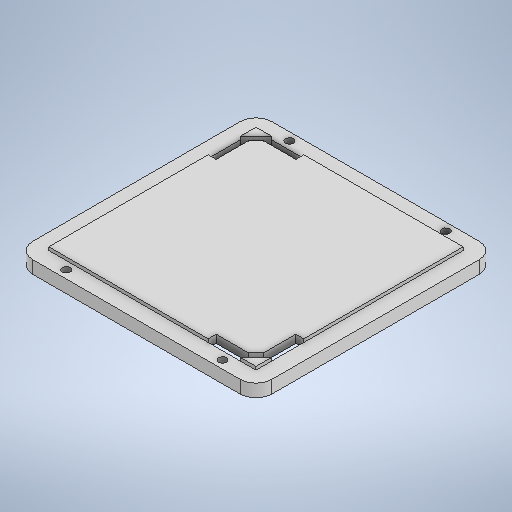
# Autodesk Inventor part: Tampa
Saved by Autodesk Inventor 2025.2 (Build 292293000, 293)
## iProperties
Created: 2025-03-23
Part Number: Tampa
Material: Genérico
Document SubType Name: Modeling
Designer: miche
Density: 1 g/cm^3
Appearance: Padrão
Author: miche
Autodesk Inventor part; units mm, degrees
ref_plane "YZ Plane" through (0, 0, 0) normal (1, 0, 0) x (0, 1, 0)
ref_plane "XZ Plane" through (0, 0, 0) normal (0, 1, 0) x (-1, 0, 0)
ref_plane "XY Plane" through (0, 0, 0) normal (0, 0, 1) x (1, 0, 0)
sketch "Esboço1" plane through (0, 0, 0) normal (0, 1, 0) x (-1, 0, 0)
  line L0 (5, 0) -> (70, 0)
  line L1 (75, -5) -> (75, -70)
  line L2 (70, -75) -> (5, -75)
  line L3 (0, -70) -> (0, -5)
  arc A0 (70, -75) -> (75, -70) centre (70, -70) ccw
  arc A1 (0, -70) -> (5, -75) centre (5, -70) ccw
  arc A2 (75, -5) -> (70, 0) centre (70, -5) ccw
  arc A3 (5, 0) -> (0, -5) centre (5, -5) ccw
  point P0 (0, 0)
  point P1 (75, -75)
  point P2 (75, 0)
  point P3 (0, -75)
  dimension "d0" = 75
  dimension "d1" = 75
  dimension "d2" = 5
  constraints: 8 end point, 8 point on circle, 8 point on line, 8 tangent, 4 centre point, 3 equal radius, 2 parallel, 1 horizontal, 1 perpendicular
  measures "d0" distance of point (75, -75) point (0, -75)
  measures "d1" distance of point (75, 0) point (75, -75)
  measures "d2" radius of A0
extrude "Extrusão1" add sketch "Esboço1" along normal blind 5
sketch "Esboço2" plane through (0, 5, 0) normal (0, 1, 0) x (1, 0, 0)
  line L0 (0, 75) -> (-13, 75)
  line L1 (-75, 75) -> (-62, 75)
  line L2 (-75, 0) -> (-62, 0)
  line L3 (-70, 0) -> (-5, 0) projected
  line L4 (0, 0) -> (-13, 0)
  line L5 (-13, 75) -> (-13, 72.5)
  line L6 (-62, 75) -> (-62, 72.5)
  line L7 (-62, 0) -> (-62, 2.5)
  line L8 (-13, 0) -> (-13, 2.5)
  circle A0 centre (-62, 72.5) radius 1.25
  circle A1 centre (-13, 72.5) radius 1.25
  circle A2 centre (-62, 2.5) radius 1.25
  circle A3 centre (-13, 2.5) radius 1.25
  dimension "d5" = 13
  dimension "d6" = 2.5
  dimension "d7" = 2.5
  dimension "d8" = 2.5
  dimension "d9" = 2.5
  dimension "d10" = 2.5
  dimension "d11" = 2.5
  constraints: 16 end point, 4 centre point, 4 coincident, 3 point on line, 3 vertical, 1 horizontal
  measures "d5" distance of L1.start L1.end
  measures "d6" distance of L0.end L5.end
  measures "d7" distance of L2.end L7.end
  measures "d8" diameter of A0
  measures "d9" diameter of A1
  measures "d10" diameter of A2
  measures "d11" diameter of A3
extrude "Extrusão2" cut sketch "Esboço2" against normal through all
sketch "Esboço3" plane through (0, 0, 0) normal (0, -1, 0) x (1, 0, 0)
  line L0 (-5, -75) -> (-70, -75) projected
  line L1 (-5, -75) -> (-5, -70)
  line L2 (-5, -70) -> (-70, -70)
  line L3 (-70, -70) -> (-70, -5)
  line L4 (-70, -5) -> (-5, -5)
  line L5 (-5, -5) -> (-5, -70)
  point P0 (0, 0)
  dimension "d14" = 5
  dimension "d15" = 65
  dimension "d16" = 65
  constraints: 10 end point, 2 parallel, 1 horizontal, 1 perpendicular, 1 vertical
  measures "d14" distance of L0.start L1.end
  measures "d15" distance of L3.end L4.end
  measures "d16" distance of L2.end L3.end
extrude "Extrusão3" cut sketch "Esboço3" against normal blind 2.5
sketch "Esboço4" plane through (0, 5, 0) normal (0, 1, 0) x (1, 0, 0)
  line L0 (-5, 70) -> (-70, 70) projected
  line L1 (-70, 70) -> (-65, 70)
  line L2 (-70, 70) -> (-70, 65)
  line L3 (-70, 65) -> (-65, 70)
  line L4 (-70, 5) -> (-5, 5) projected
  line L5 (-5, 5) -> (-5, 10)
  line L6 (-5, 5) -> (-5, 70) projected
  line L7 (-5, 5) -> (-10, 5)
  line L8 (-10, 5) -> (-5, 10)
  line L9 (-70, 65) -> (-70, 55)
  line L10 (-70, 70) -> (-70, 5) projected
  line L11 (-70, 55) -> (-67.5, 55)
  line L12 (-65, 70) -> (-55, 70)
  line L13 (-55, 70) -> (-55, 67.5)
  line L14 (-55, 67.5) -> (-63.9645, 67.5)
  line L15 (-65, 70) -> (-55, 70)
  line L16 (-70, 65) -> (-70, 55)
  line L17 (-67.5, 65) -> (-65, 67.5)
  line L18 (-67.5, 65) -> (-67.5, 55)
  line L19 (-65, 67.5) -> (-63.9645, 67.5)
  point P0 (0, 0)
  constraints: 32 end point, 5 point on line, 3 vertical, 2 horizontal, 2 perpendicular, 1 collinear
sketch "Esboço5" plane through (0, 5, 0) normal (0, 1, 0) x (1, 0, 0)
  line L0 (-5, 5) -> (-5, 70) projected
  line L1 (-5, 10) -> (-5, 20)
  line L2 (-5, 20) -> (-7.5, 20)
  line L3 (-70, 5) -> (-5, 5) projected
  line L4 (-10, 5) -> (-20, 5)
  line L5 (-20, 5) -> (-20, 7.5)
  line L6 (-7.5, 10) -> (-10, 7.5)
  line L7 (-7.5, 20) -> (-7.5, 10)
  line L8 (-20, 7.5) -> (-10, 7.5)
  line L9 (-5, 20) -> (-5, 10)
  line L10 (-20, 5) -> (-10, 5)
  line L11 (-10, 5) -> (-5, 10)
  point P0 (0, 0)
  dimension "d23" = 2.5
  dimension "d24" = 10
  dimension "d25" = 2.5
  constraints: 20 end point, 4 point on line, 3 perpendicular, 1 collinear, 1 vertical
  measures "d23" distance of L1.end L2.end
  measures "d24" distance of L4.start L4.end
  measures "d25" distance of L4.end L5.end
extrude "Extrusão4" cut sketch "Esboço5" against normal through all contours L11 L3 L5 L8 L6 L7 L2 L0
extrude "Extrusão5" cut sketch "Esboço4" against normal through all contours L13 L14 L19 L17 L18 L11 L9 L3 L0
sketch "Esboço6" plane through (0, 5, 0) normal (0, 1, 0) x (1, 0, 0)
  line L0 (-70, 70) -> (-70, 5) projected
  line L1 (-5, 5) -> (-5, 70) projected
  line L2 (-70, 70) -> (-5, 70)
  line L3 (-5, 70) -> (-5, 5)
  line L4 (-5, 5) -> (-70, 5)
  line L5 (-70, 5) -> (-70, 70)
  arc A0 (0, 70) -> (-5, 75) centre (-5, 70) ccw projected
  line L6 (-5, 75) -> (0, 75)
  line L7 (0, 75) -> (0, 0)
  line L8 (0, 0) -> (-5, 0)
  line L9 (-5, 0) -> (-5, 75)
  line L10 (-75, 75) -> (0, 75)
  line L11 (0, 75) -> (0, 70)
  line L12 (0, 70) -> (-75, 70)
  line L13 (-75, 70) -> (-75, 75)
  line L14 (0, 0) -> (-75, 0)
  line L15 (-75, 0) -> (-75, 5)
  line L16 (-75, 5) -> (0, 5)
  line L17 (0, 5) -> (0, 0)
  line L18 (-75, 0) -> (-70, 0)
  line L19 (-70, 0) -> (-70, 75)
  line L20 (-70, 75) -> (-75, 75)
  line L21 (-75, 75) -> (-75, 0)
  constraints: 40 end point, 10 parallel, 6 point on line, 5 horizontal, 5 perpendicular
extrude "Extrusão6" cut sketch "Esboço6" against normal blind 1 contours L19 L10 L9 L2 | L0 L16 L21 L12 | L12 L13 L10 L19 | L19 L14 L15 L16 | L4 L9 L14 L19 | L12 L7 L16 L1 | L9 A0 L12 | L16 L7 L8 L9 | L6 L7 A0
thread "Rosca1" size "M2.5x0.45" class "6H" standard "ANSI Metric M Profile" length 11
thread "Rosca2" size "M2.5x0.45" class "6H" standard "ANSI Metric M Profile" length 11
thread "Rosca3" size "M2.5x0.45" class "6H" standard "ANSI Metric M Profile" length 11
thread "Rosca4" size "M2.5x0.45" class "6H" standard "ANSI Metric M Profile" length 11
